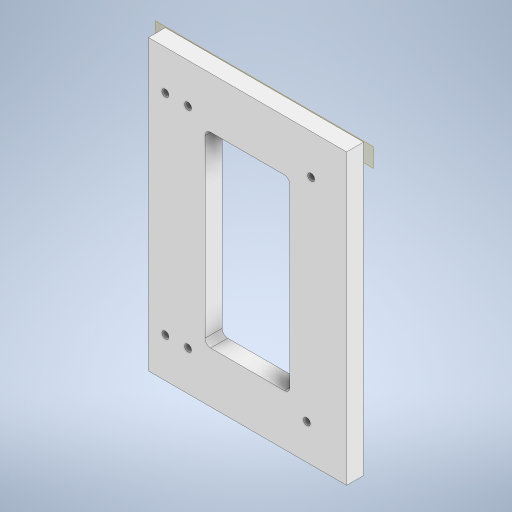
# Autodesk Inventor part: 62
Saved by Autodesk Inventor 2024.3 (Build 283343000, 343)
## iProperties
Created: 2024-09-09
Part Number: 62
Material: 아크릴, 선명
Document SubType Name: Modeling
Designer: 구지현
Density: 1.19 g/cm^3
Appearance: 흰색
Author: 구지현
Autodesk Inventor part; units mm, degrees
ref_plane "YZ Plane" through (0, 0, 0) normal (1, 0, 0) x (0, 1, 0)
ref_plane "XZ Plane" through (0, 0, 0) normal (0, 1, 0) x (-1, 0, 0)
ref_plane "XY Plane" through (0, 0, 0) normal (0, 0, 1) x (1, 0, 0)
ref_plane "작업 평면1" through (-67, 45, 0) normal (0, 0, 1) x (1, 0, 0)
sketch "스케치1" plane through (-67, 45, 0) normal (0, 0, 1) x (1, 0, 0)
  line L0 (0, 0) -> (70, 0) projected
  line L1 (70, 0) -> (70, 6) projected
  line L2 (0, 6) -> (70, 6) projected
  line L3 (0, 0) -> (0, 6) projected
  line L4 (70, 0) -> (64, 0) projected
  line L5 (64, 0) -> (64, -90) projected
  line L6 (64, -90) -> (70, -90) projected
  line L7 (70, -90) -> (70, 0) projected
  line L8 (70, -90) -> (0, -90) projected
  line L9 (0, -90) -> (0, -96) projected
  line L10 (70, -96) -> (0, -96) projected
  line L11 (70, -90) -> (70, -96) projected
  line L12 (70, 6) -> (0, 6)
  line L13 (0, 6) -> (0, -96)
  line L14 (0, -96) -> (70, -96)
  line L15 (70, -96) -> (70, 6)
  point P0 (67, -45)
  constraints: 8 end point, 2 parallel, 1 horizontal, 1 perpendicular
extrude "돌출1" add sketch "스케치1" along normal blind 6
sketch "스케치2" plane through (-67, 45, 6) normal (0, 0, 1) x (1, 0, 0)
  circle A0 centre (6, -8) radius 1.25 projected
  circle A1 centre (14, -8) radius 1.25 projected
  line L0 (20, -3) -> (0, -3) projected
  line L1 (20, -3) -> (20, -13) projected
  line L2 (0, -13) -> (20, -13) projected
  line L3 (0, -3) -> (0, -13) projected
  circle A2 centre (57.5, -8) radius 1.25 projected
  line L4 (61, -13) -> (61, -3) projected
  line L5 (54, -13) -> (61, -13) projected
  line L6 (54, -3) -> (54, -13) projected
  line L7 (61, -3) -> (54, -3) projected
  circle A3 centre (56, -83.5) radius 1.25 projected
  line L8 (51, -87) -> (61, -87) projected
  line L9 (51, -80) -> (51, -87) projected
  line L10 (61, -80) -> (51, -80) projected
  line L11 (61, -87) -> (61, -80) projected
  circle A4 centre (14, -82) radius 1.25 projected
  circle A5 centre (6, -82) radius 1.25 projected
  line L12 (0, -87) -> (20, -87) projected
  line L13 (0, -87) -> (0, -77) projected
  line L14 (20, -77) -> (0, -77) projected
  line L15 (20, -87) -> (20, -77) projected
  point P0 (67, -45)
extrude "돌출2" cut sketch "스케치2" against normal blind 6 contours A0 | A1 | A2 | A3 | A4 | A5
sketch "스케치3" plane through (-67, 45, 6) normal (0, 0, 1) x (1, 0, 0)
  circle A0 centre (57.5, -8) radius 1.25 projected
  circle A1 centre (6, -82) radius 1.25 projected
  circle A2 centre (14, -8) radius 1.25 projected
  circle A3 centre (56, -83.5) radius 1.25 projected
  circle A4 centre (14, -82) radius 1.25 projected
  circle A5 centre (6, -8) radius 1.25 projected
  line L0 (0, 6) -> (0, -96) projected
  line L1 (0, -96) -> (70, -96) projected
  line L2 (70, -96) -> (70, 6) projected
  line L3 (70, 6) -> (0, 6) projected
  line L4 (70, -96) -> (70, 6) projected
  line L5 (0, 6) -> (0, -96) projected
  line L6 (0, -96) -> (70, -96) projected
  line L7 (70, 6) -> (0, 6) projected
  line L8 (20, -78) -> (50, -78)
  line L9 (50, -78) -> (50, -12)
  line L10 (50, -12) -> (20, -12)
  line L11 (20, -12) -> (20, -78)
  point P0 (67, -45)
  point P1 (50, -64.8252)
  point P2 (20, -61.3274)
  point P3 (30.9806, -78)
  point P4 (28.8515, -12)
  point P5 (28.8515, -12)
  dimension "d4" = 20
  dimension "d5" = 20
  dimension "d6" = 18
  dimension "d7" = 18
  constraints: 8 end point, 2 parallel, 1 coincident, 1 horizontal, 1 perpendicular
  measures "d4" distance from line of L4 point (50, -64.825)
  measures "d5" distance from line of point (20, -61.327) L5
  measures "d6" distance from line of L6 point (30.981, -78)
  measures "d7" distance from line of L7 point (28.851, -12)
extrude "돌출3" cut sketch "스케치3" against normal blind 6 contours L11 L10 L9 L8
fillet "모깎기1" radius 2 4 edges at (-47, -33, 3) (-17, -33, 3) (-47, 33, 3) (-17, 33, 3)
